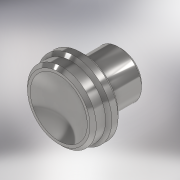
# Autodesk Inventor part: 钢珠定位圈
Saved by Autodesk Inventor 2020 (Build 240168000, 168)
## iProperties
Created: 2021-04-21
Part Number: 钢珠定位圈
Material: 钢
Document SubType Name: Modeling
Designer: Luorily
Density: 7.85 g/cm^3
Appearance: 钢 - 抛光
Author: Luorily
Autodesk Inventor part; units mm, degrees
ref_plane "YZ Plane" through (0, 0, 0) normal (1, 0, 0) x (0, 1, 0)
ref_plane "XZ Plane" through (0, 0, 0) normal (0, 1, 0) x (-1, 0, 0)
ref_plane "XY Plane" through (0, 0, 0) normal (0, 0, 1) x (1, 0, 0)
sketch "草图1" plane through (0, 0, 0) normal (0, 0, 1) x (1, 0, 0)
  circle A0 centre (0, 0) radius 6
  dimension "d0" = 12
  constraints: 1 centre point, 1 coincident
  measures "d0" diameter of A0
extrude "拉伸1" add sketch "草图1" along normal blind 2
sketch "草图2" plane through (0, 0, 2) normal (0, 0, 1) x (1, 0, 0)
  circle A0 centre (0, 0) radius 6 projected
  circle A1 centre (0, 0) radius 5.5
  dimension "d3" = 11
  constraints: 1 centre point, 1 coincident
  measures "d3" diameter of A1
extrude "拉伸2" add sketch "草图2" along normal blind 2 contours A1
sketch "草图3" plane through (0, 0, 0) normal (0, 0, -1) x (-1, 0, 0)
  circle A0 centre (0, 0) radius 6 projected
  circle A1 centre (0, 0) radius 3.75
  dimension "d6" = 7.5
  constraints: 1 centre point, 1 coincident
  measures "d6" diameter of A1
extrude "拉伸3" add sketch "草图3" along normal blind 6 contours A1
sketch "草图4" plane through (0, 0, 0) normal (0, 1, 0) x (-1, 0, 0)
  line L0 (6, 2) -> (-6, 2) projected
  arc A0 (0, 14.4) -> (0, 2) centre (0, 8.2) ccw
  line L1 (0, 2) -> (0, 14.4)
  point P0 (0, 0)
  constraints: 2 end point, 2 point on circle, 1 centre point, 1 midpoint, 1 perpendicular
revolve "旋转1" cut sketch "草图4" angle 360 about axis through (0, 0, 2) along (0, 0, 1)
chamfer "倒角1" distance 0.5 angle 45 4 edges at (3.75, 0, -6) (-6, 0, 0) (-6, 0, 2) (-5.5, 0, 4)
